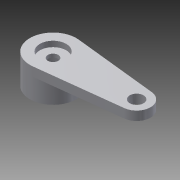
# Autodesk Inventor part: Servo Arm
Saved by Autodesk Inventor 2013 (Build 170138000, 138)
## iProperties
Created: 2012-10-29
Part Number: Servo Arm
Material: Generic
Document SubType Name: Modeling
Designer: uqgtayle
Density: 1 g/cm^3
Author: uqgtayle
Autodesk Inventor part; units mm, degrees
ref_plane "YZ Plane" through (0, 0, 0) normal (1, 0, 0) x (0, 1, 0)
ref_plane "XZ Plane" through (0, 0, 0) normal (0, 1, 0) x (-1, 0, 0)
ref_plane "XY Plane" through (0, 0, 0) normal (0, 0, 1) x (1, 0, 0)
sketch "Sketch1" plane through (0, 0, 0) normal (0, 0, 1) x (1, 0, 0)
  arc A0 (0.3627, 3.3303) -> (0.3911, -3.3271) centre (0, 0) ccw
  arc A1 (12.2334, -1.9351) -> (12.2164, 2.0395) centre (11.9999, 0.0513) ccw
  line L0 (0.3627, 3.3303) -> (12.2164, 2.0395)
  line L1 (12.2334, -1.9351) -> (0.3911, -3.3271)
  dimension "d0" = 6.7
  dimension "d2" = 4
  dimension "d3" = 12
  constraints: 4 end point, 4 point on circle, 4 tangent, 2 centre point, 1 coincident
  measures "d0" diameter of A0
  measures "d2" diameter of A1
  measures "d3" distance of A1.centre point (0, 0)
extrude "Extrusion1" add sketch "Sketch1" against normal blind 1.3
sketch "Sketch2" plane through (0, 0, -1.3) normal (0, 0, -1) x (-1, 0, 0)
  arc A0 (-0.3911, -3.3271) -> (-0.3627, 3.3303) centre (0, 0) ccw projected
  circle A1 centre (0, 0) radius 3.35
  dimension "d6" = 6.7
  constraints: 1 centre point, 1 coincident
  measures "d6" diameter of A1
extrude "Extrusion2" add sketch "Sketch2" along normal blind 3
sketch "Sketch3" plane through (0, 0, 0) normal (0, 0, 1) x (1, 0, 0)
  arc A0 (0.3627, 3.3303) -> (0.3911, -3.3271) centre (0, 0) ccw projected
  constraints: 1 coincident
hole "Hole1" at (0, 0, 0) direction (0, 0, -1) diameter 1.5 end through all counterbore diameter 3.8 counterbore depth 0.8
sketch "Sketch4" plane through (0, 0, -4.3) normal (0, 0, -1) x (-1, 0, 0)
  circle A0 centre (0, 0) radius 0.75 projected
  circle A1 centre (0, 0) radius 3.35 projected
  circle A2 centre (0, 0) radius 2
  dimension "d17" = 4
  constraints: 1 centre point, 1 coincident
  measures "d17" diameter of A2
extrude "Extrusion3" cut sketch "Sketch4" against normal blind 3 contours A2
sketch "Sketch5" plane through (0, 0, 0) normal (0, 0, 1) x (1, 0, 0)
  arc A0 (12.2334, -1.9351) -> (12.2164, 2.0395) centre (11.9999, 0.0513) ccw projected
  constraints: 1 coincident
hole "Hole2" at (11.9999, 0.0513, 0) direction (0, 0, -1) diameter 2 end through all
body "Solid1"
